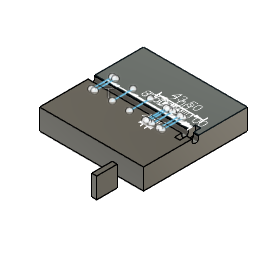
Tube+Cutter (Autodesk Fusion 360 design; units mm, degrees)
Autodesk Fusion 360 part; units mm, degrees
sketch "Sketch1" plane through (0, 0, 0) normal (0, 0, 1) x (1, 0, 0)
  line L0 (0, 0) -> (-100, 0)
  line L1 (-100, 0) -> (-100, 100)
  line L2 (-100, 100) -> (0, 100)
  line L3 (0, 100) -> (0, 0)
  line L4 (-20, -10) -> (-15.2, -10)
  line L5 (-15.2, -10) -> (-15.2, -29.8)
  line L6 (-15.2, -29.8) -> (-20, -29.8)
  line L7 (-20, -29.8) -> (-20, -10)
  dimension "d11" = 4.8
  dimension "d12" = 19.8
  constraint horizontal L0
  constraint vertical L1
  constraint horizontal L2
  constraint vertical L3
  constraint coincident L0.start L3.end
  constraint horizontal L4
  constraint vertical L5
  constraint horizontal L6
  constraint vertical L7
  measures "d11" distance of L4.start L4.end
  measures "d12" distance of L4.start L6.end
extrude "Extrude1" add sketch "Sketch1" along normal blind 20 contours L0 L1 L2 L3 makes body 1
sketch "Sketch2" plane through (-100, 0, 0) normal (-1, 0, 0) x (0, -1, 0)
  line L0 (-100, 0) -> (0, 0)
  line L1 (0, 0) -> (0, 20)
  line L2 (0, 20) -> (-100, 20)
  line L3 (-100, 20) -> (-100, 0)
  circle A0 centre (-50, 18) radius 3.2
  line L4 (-50, 18) -> (-53.2, 18)
  line L5 (-50, 18) -> (-46.8, 18)
  line L6 (-53.2, 18) -> (-46.8, 18)
  line L7 (-46.8, 18) -> (-46.8, 20)
  line L8 (-46.8, 20) -> (-53.2, 20)
  line L9 (-53.2, 20) -> (-53.2, 18)
  dimension "d3" = 6.4
  constraint coincident A0.centre L4.start
  constraint coincident A0 L4.end
  constraint horizontal L4
  constraint coincident A0 L5.end
  constraint parallel L4 L5
  constraint horizontal L6
  constraint vertical L7
  constraint horizontal L8
  constraint vertical L9
  constraint coincident L2 L7.end
  measures "d3" diameter of A0
extrude "Extrude2" cut sketch "Sketch2" against normal blind 115 contours L2 A0 L8 | L2 A0 L4 L5 L6 L8 | A0 L4 L5 L6 bodies 1
fillet "Fillet1" radius 0.5 2 edges at (-50, 52.498, 20) (-50, 47.502, 20) on bodies 1
sketch "Sketch3" plane through (0, 0, 20) normal (0, 0, 1) x (-1, 0, 0)
  line L0 (100, -53.3823) -> (0, -53.3823)
  line L1 (0, -53.3823) -> (0, -100)
  line L2 (0, -100) -> (100, -100)
  line L3 (100, -100) -> (100, -53.3823)
  line L4 (10, -60) -> (5, -60)
  line L5 (5, -60) -> (5, -40)
  line L6 (5, -40) -> (10, -40)
  line L7 (10, -40) -> (10, -60)
  constraint horizontal L4
  constraint vertical L5
  constraint horizontal L6
  constraint vertical L7
extrude "Extrude3" cut sketch "Sketch3" against normal blind 8 contours L0 L4 L5 L7 | L0 L5 L6 L7 bodies 1
extrude "Extrude4" add sketch "Sketch1" along normal blind 19.8 separate body contours L4 L5 L6 L7 makes body 2
sketch "Sketch4" plane through (0, 0, 20) normal (0, 0, 1) x (-1, 0, 0)
  line L0 (5, -60) -> (5, -53.3823)
  line L1 (5, -53.3823) -> (0, -53.3823)
  line L2 (0, -53.3823) -> (0, -100)
  line L3 (0, -100) -> (100, -100)
  line L4 (100, -100) -> (100, -53.3823)
  line L5 (100, -53.3823) -> (10, -53.3823)
  line L6 (10, -53.3823) -> (10, -60)
  line L7 (10, -60) -> (5, -60)
  line L8 (22, -60) -> (22, -40)
  line L9 (25, -40) -> (25, -60)
  line L10 (32, -60) -> (32, -40)
  line L11 (36, -40) -> (36, -60)
  line L12 (38, -60) -> (38, -40)
  line L13 (53.5, -60) -> (53.5, -40)
  line L14 (70, -60) -> (70, -40)
  line L15 (90, -60) -> (90, -40)
  line L16 (87, -60) -> (87, -40)
  dimension "d15" = 12
  dimension "d16" = 7
  dimension "d17" = 4
  dimension "d18" = 2
  dimension "d19" = 43.5
  dimension "d20" = 60
  dimension "d21" = 80
  dimension "d22" = 77
  constraint perpendicular L5 L16
  measures "d15" distance of L6.end L8.start
  measures "d16" distance of L9.end L10.start
  measures "d17" distance of L10.end L11.start
  measures "d18" distance of L11.end L12.start
  measures "d19" distance of L6.end L13.start
  measures "d20" distance of L6.end L14.start
  measures "d21" distance of L6.end L15.start
  measures "d22" distance of L6.end L16.start
